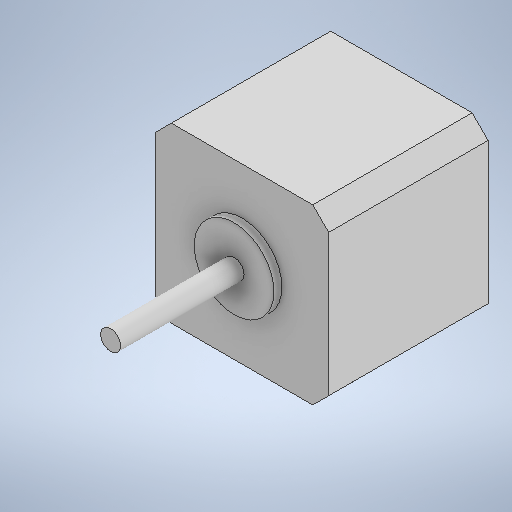
# Autodesk Inventor part: Stepper Simulation
Saved by Autodesk Inventor 2025.4 (Build 294407000, 407)
## iProperties
Created: 2026-04-04
Part Number: Stepper Simulation
Material: Generic
Document SubType Name: Modeling
Designer: lenovo
Density: 1 g/cm^3
Appearance: Default
Author: lenovo
Autodesk Inventor part; units mm, degrees
ref_plane "YZ Plane" through (0, 0, 0) normal (1, 0, 0) x (0, 1, 0)
ref_plane "XZ Plane" through (0, 0, 0) normal (0, 1, 0) x (-1, 0, 0)
ref_plane "XY Plane" through (0, 0, 0) normal (0, 0, 1) x (1, 0, 0)
sketch "Sketch1" plane through (0, 0, 0) normal (0, 0, 1) x (1, 0, 0)
  line L0 (-21.75, -21.75) -> (21.75, -21.75)
  line L1 (21.75, -21.75) -> (21.75, 21.75)
  line L2 (21.75, 21.75) -> (-21.75, 21.75)
  line L3 (-21.75, 21.75) -> (-21.75, -21.75)
  line L4 (-21.75, -21.75) -> (21.75, 21.75) construction
  line L5 (21.75, -21.75) -> (-21.75, 21.75) construction
  point P0 (0, 0)
  dimension "d0" = 43.5
  constraints: 12 end point, 2 midpoint, 2 parallel, 2 perpendicular, 1 horizontal
  measures "d0" distance of L1.end L2.end
extrude "Extrusion1" add sketch "Sketch1" along normal blind 40
sketch "Sketch2" plane through (0, 0, 40) normal (0, 0, 1) x (1, 0, 0)
  circle A0 centre (0, 0) radius 10
  dimension "d3" = 20
  constraints: 1 centre point, 1 coincident
  measures "d3" diameter of A0
extrude "Extrusion2" add sketch "Sketch2" along normal blind 2
sketch "Sketch3" plane through (0, 0, 42) normal (0, 0, 1) x (1, 0, 0)
  circle A0 centre (0, 0) radius 2.5
  dimension "d6" = 5
  constraints: 1 centre point, 1 coincident
  measures "d6" diameter of A0
extrude "Extrusion3" add sketch "Sketch3" along normal blind 31
chamfer "Chamfer1" distance 4 angle 45 4 edges at (21.75, 21.75, 20) (-21.75, 21.75, 20) (21.75, -21.75, 20) (-21.75, -21.75, 20)
body "Solid1"
